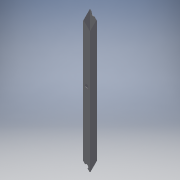
# Autodesk Inventor part: AP 4
Saved by Autodesk Inventor 2016 (Build 200138000, 138)
## iProperties
Created: 2016-02-17
Part Number: AP 4
Material: Generic
Document SubType Name: Modeling
Designer: Admin
Density: 1 g/cm^3
Appearance: Default
Author: Admin
Autodesk Inventor part; units mm, degrees
ref_plane "YZ Plane" through (0, 0, 0) normal (1, 0, 0) x (0, 1, 0)
ref_plane "XZ Plane" through (0, 0, 0) normal (0, 1, 0) x (-1, 0, 0)
ref_plane "XY Plane" through (0, 0, 0) normal (0, 0, 1) x (1, 0, 0)
sketch "Sketch1" plane through (0, 0, 0) normal (0, 1, 0) x (-1, 0, 0)
  line L0 (0, 0) -> (25.4, 0)
  line L1 (25.4, 0) -> (25.4, -25.4)
  line L2 (25.4, -25.4) -> (0, -25.4)
  line L3 (0, -25.4) -> (0, 0)
  line L4 (23.8125, -23.8125) -> (23.8125, -1.5875)
  line L5 (23.8125, -1.5875) -> (1.5875, -1.5875)
  line L6 (1.5875, -1.5875) -> (1.5875, -23.8125)
  line L7 (1.5875, -23.8125) -> (23.8125, -23.8125)
  dimension "d0" = 25.4
  dimension "d1" = 25.4
  dimension "d2" = 1.5875
  constraints: 16 end point, 4 parallel, 2 perpendicular, 1 horizontal, 3 other
  measures "d0" distance of L1.end L2.end
  measures "d1" distance of L0.end L1.end
  measures "d2" distance between parallel lines of L1 L4
extrude "Extrusion1" add sketch "Sketch1" along normal blind 405.9428
sketch "Sketch4" plane through (-25.4, 0, 0) normal (0, 0, 1) x (1, 0, 0)
  circle A0 centre (12.7, 177.8) radius 6.35
  line L0 (0, 0) -> (0, 405.9428) projected
  line L1 (25.4, 0) -> (0, 0) projected
  dimension "d13" = 12.7
  dimension "d14" = 12.7
  dimension "d15" = 177.8
  constraints: 1 centre point
  measures "d13" diameter of A0
  measures "d14" distance from line of A0.centre L0
  measures "d15" distance from line of L1 A0.centre
extrude "Extrusion4" cut sketch "Sketch4" against normal blind 25.4
sketch "Sketch5" plane through (0, 0, 0) normal (0, -1, 0) x (1, 0, 0)
  line L0 (-25.4, -25.4) -> (0, -25.4) projected
  line L1 (0, 0) -> (-25.4, 0) projected
  line L2 (-25.4, -25.4) -> (0, -25.4)
  line L3 (0, -25.4) -> (0, 0)
  line L4 (0, 0) -> (-25.4, 0)
  line L5 (-25.4, 0) -> (-25.4, -25.4)
  line L6 (-23.8125, -1.5875) -> (-1.5875, -1.5875) projected
  line L7 (-23.8125, -23.8125) -> (-23.8125, -1.5875) projected
  line L8 (-1.5875, -1.5875) -> (-23.8125, -1.5875)
  line L9 (-23.8125, -1.5875) -> (-23.8125, -23.8125)
  line L10 (-23.8125, -23.8125) -> (-1.5875, -23.8125)
  line L11 (-1.5875, -23.8125) -> (-1.5875, -1.5875)
  constraints: 16 end point, 4 parallel, 2 horizontal, 2 perpendicular
extrude "Extrusion5" add sketch "Sketch5" along normal blind 38.1
sketch "Sketch6" plane through (-25.4, 405.9428, 0) normal (0, 0, 1) x (1, 0, 0)
  circle A0 centre (12.7, -431.3428) radius 6.35
  line L0 (25.4, -444.0428) -> (0, -444.0428) projected
  line L1 (0, 0) -> (0, -444.0428) projected
  point P0 (25.4, -405.9428)
  dimension "d21" = 12.7
  dimension "d22" = 12.7
  dimension "d23" = 12.7
  constraints: 1 centre point
  measures "d21" diameter of A0
  measures "d22" distance from line of A0.centre L0
  measures "d23" distance from line of L1 A0.centre
extrude "Extrusion6" cut sketch "Sketch6" against normal blind 38.1
sketch "Sketch7" plane through (0, 405.9428, -25.4) normal (0, 0, -1) x (-1, 0, 0)
  circle A0 centre (12.7, -12.7) radius 6.35
  line L0 (0, 0) -> (0, -444.0428) projected
  line L1 (25.4, -444.0428) -> (0, -444.0428) projected
  line L2 (0, 0) -> (25.4, 0) projected
  point P0 (0, -405.9428)
  dimension "d26" = 12.7
  dimension "d31" = 12.7
  dimension "d32" = 12.7
  constraints: 1 centre point
  measures "d26" diameter of A0
  measures "d31" distance from line of L0 A0.centre
  measures "d32" distance from line of L2 A0.centre
extrude "Extrusion7" cut sketch "Sketch7" against normal blind 25.4
body "Solid1"
